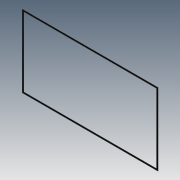
# Autodesk Inventor part: GE-12017-01
Saved by Autodesk Inventor 2012 (Build 160160000, 160)
## iProperties
Created: 2011-11-18
Part Number: GE-12017-01
Document SubType Name: Modeling
Designer: dfoster
Density: 1 g/cm^3
Mass: 272.435 g
Surface Area: 3646.77 cm^2
Volume: 272.435 cm^3
Material: Default
Title: 1" Hook Velcro, Adhesive Backed, 266" total
Author: dfoster
Autodesk Inventor part; units mm, degrees
ref_plane "YZ Plane" through (0, 0, 0) normal (1, 0, 0) x (0, 1, 0)
ref_plane "XZ Plane" through (0, 0, 0) normal (0, 1, 0) x (-1, 0, 0)
ref_plane "XY Plane" through (0, 0, 0) normal (0, 0, 1) x (1, 0, 0)
sketch "Sketch1" plane through (0, 0, 0) normal (0, 0, 1) x (1, 0, 0)
  line L0 (0, 0) -> (2235.2, 0)
  line L1 (2235.2, 0) -> (2235.2, -1193.8)
  line L2 (2235.2, -1193.8) -> (0, -1193.8)
  line L3 (0, -1193.8) -> (0, 0)
  line L4 (2209.8, -25.4) -> (25.4, -25.4)
  line L5 (25.4, -25.4) -> (25.4, -1168.4)
  line L6 (25.4, -1168.4) -> (2209.8, -1168.4)
  line L7 (2209.8, -1168.4) -> (2209.8, -25.4)
  dimension "d0" = 2235.2
  dimension "d1" = 1193.8
  dimension "d2" = 25.4
  constraints: 16 end point, 3 other
  measures "d0" distance of L0.start L0.end
  measures "d1" distance of L2.end L0.start
  measures "d2" distance between parallel lines of L0 L4
extrude "Extrusion1" add sketch "Sketch1" along normal blind 1.5875
body "Solid1"
